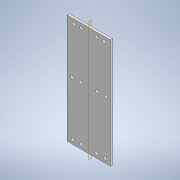
# Autodesk Inventor part: body_bone_1
Saved by Autodesk Inventor 2020 (Build 240168000, 168)
## iProperties
Created: 2019-05-16
Part Number: body_bone_1
Material: Generic
Document SubType Name: Modeling
Designer: psrob
Density: 1 g/cm^3
Appearance: Default
Author: psrob
Autodesk Inventor part; units mm, degrees
ref_plane "YZ Plane" through (0, 0, 0) normal (1, 0, 0) x (0, 1, 0)
ref_plane "XZ Plane" through (0, 0, 0) normal (0, 1, 0) x (-1, 0, 0)
ref_plane "XY Plane" through (0, 0, 0) normal (0, 0, 1) x (1, 0, 0)
sketch "Sketch1" plane through (0, 0, 0) normal (0, 0, 1) x (1, 0, 0)
  circle A0 centre (-11, -99.1166) radius 1.5 projected
  circle A1 centre (-13, -89.1166) radius 1.5 projected
  circle A2 centre (-5, -89.1166) radius 1.5 projected
  line L0 (0, -100.499) -> (0, -85.1166) projected
  line L1 (0, -85.1166) -> (-20, -85.1166) projected
  line L2 (-20, -85.1166) -> (-20, -111.0877) projected
  line L3 (-20, -111.0877) -> (-11.9783, -111.0877) projected
  line L4 (-11.9783, -111.0877) -> (-7.95, -105.7166) projected
  arc A3 (0, -100.499) -> (-7.95, -105.7166) centre (3.25, -114.1166) ccw projected
  circle A4 centre (-29, -99.1166) radius 1.5 projected
  circle A5 centre (-27, -89.1166) radius 1.5 projected
  circle A6 centre (-35, -89.1166) radius 1.5 projected
  line L5 (-40, -100.499) -> (-40, -85.1166) projected
  arc A7 (-32.05, -105.7166) -> (-40, -100.499) centre (-43.25, -114.1166) ccw projected
  line L6 (-28.0217, -111.0877) -> (-32.05, -105.7166) projected
  line L7 (-20, -111.0877) -> (-28.0217, -111.0877) projected
  line L8 (-20, -85.1166) -> (-20, -111.0877) projected
  line L9 (-40, -85.1166) -> (-20, -85.1166) projected
  circle A8 centre (-6, 4) radius 1.5 projected
  circle A9 centre (-10, 13) radius 1.5 projected
  circle A10 centre (-13, 4) radius 1.5 projected
  line L10 (-10, 23) -> (-10, 40) projected
  line L11 (-20, 40) -> (-10, 40) projected
  line L12 (-20, 0) -> (-20, 40) projected
  line L13 (0, 0) -> (-20, 0) projected
  line L14 (0, 0) -> (0, 8) projected
  line L15 (0, 8) -> (-10, 23) projected
  circle A11 centre (-34, 4) radius 1.5 projected
  circle A12 centre (-30, 13) radius 1.5 projected
  circle A13 centre (-27, 4) radius 1.5 projected
  line L16 (-30, 23) -> (-30, 40) projected
  line L17 (-40, 8) -> (-30, 23) projected
  line L18 (-40, 0) -> (-40, 8) projected
  line L19 (-40, 0) -> (-20, 0) projected
  line L20 (-20, 0) -> (-20, 40) projected
  line L21 (-20, 40) -> (-30, 40) projected
  line L22 (0, 0) -> (-40, 0)
  line L23 (-40, 0) -> (-40, 8)
  line L24 (-40, 8) -> (0, 8)
  line L25 (0, 8) -> (0, 0)
  line L26 (0, -85.1166) -> (-40, -85.1166)
  line L27 (-40, -85.1166) -> (-40, -93.1166)
  line L28 (-40, -93.1166) -> (0, -93.1166)
  line L29 (0, -93.1166) -> (0, -85.1166)
  line L30 (0, -85.1166) -> (-40, -85.1166)
  line L31 (-40, -85.1166) -> (-40, 0)
  line L32 (-40, 0) -> (0, 0)
  line L33 (0, 0) -> (0, -85.1166)
  point P0 (0, -93.1166)
  dimension "d0" = 40
  dimension "d1" = 8
  dimension "d2" = 40
  dimension "d3" = 8
  constraints: 24 end point, 6 parallel, 3 horizontal, 3 perpendicular
  measures "d0" distance of L17.start L24.end
  measures "d1" distance of L22.end L17.start
  measures "d2" distance of L28.end L27.end
  measures "d3" distance of L27.end L26.end
extrude "Extrusion1" add sketch "Sketch1" along normal blind 2 contours L28 L2 L1 L0 | L1 L9 L31 L19 L13 L33 | L28 L5 L9 L2 | L13 L12 L24 L14 | L19 L18 L24 L12
sketch "Sketch2" plane through (0, 0, 0) normal (0, 0, -1) x (-1, 0, 0)
  circle A0 centre (12.2614, -39.5) radius 1.5 projected
  circle A1 centre (4.2614, -39.5) radius 1.5 projected
  point P0 (0, 0)
extrude "Extrusion2" cut sketch "Sketch2" against normal blind 10
ref_plane "Work Plane1" through (-20, -93.1166, 0) normal (1, 0, 0) x (0, 0, -1)
mirror "Mirror1" about plane through (-20, -93.1166, 0) normal (1, 0, 0) of "Extrusion2"
body "Solid1"
